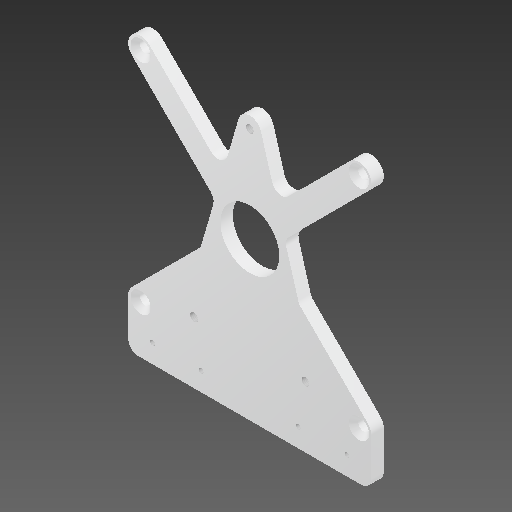
# Autodesk Inventor part: motor_support
Saved by Autodesk Inventor 2020.2 (Build 242310000, 310)
## iProperties
Created: 2020-03-23
Part Number: motor_support
Material: Aluminum 6061
Document SubType Name: Modeling
Designer: agmle
Density: 2.7 g/cm^3
Appearance: Aluminum - Flat
Mass: 160.03 g
Surface Area: 243.177 cm^2
Volume: 59.2703 cm^3
Author: agmle
Autodesk Inventor part; units mm, degrees
ref_plane "YZ Plane" through (0, 0, 0) normal (1, 0, 0) x (0, 1, 0)
ref_plane "XZ Plane" through (0, 0, 0) normal (0, 1, 0) x (-1, 0, 0)
ref_plane "XY Plane" through (0, 0, 0) normal (0, 0, 1) x (1, 0, 0)
sketch "Sketch1" plane through (0, 0, 0) normal (0, 0, 1) x (1, 0, 0)
  line L0 (36.3099, 124.6816) -> (0, 0)
  line L1 (0, 0) -> (72.6199, 0)
  line L2 (72.6199, 0) -> (36.3099, 124.6816)
  circle A0 centre (36.3099, 103.4017) radius 5.95 construction
  circle A1 centre (7.9299, 5.95) radius 5.95 construction
  circle A2 centre (64.6899, 5.95) radius 5.95 construction
  line L3 (36.3099, 103.4017) -> (7.9299, 5.95) construction
  line L4 (7.9299, 5.95) -> (64.6899, 5.95) construction
  line L5 (64.6899, 5.95) -> (36.3099, 103.4017) construction
  circle A3 centre (36.3098, 54.6757) radius 15
  line L6 (36.3099, 103.4017) -> (36.3098, 54.6757) construction
  line L7 (36.3098, 54.6757) -> (7.9299, 5.95) construction
  line L8 (36.3098, 54.6757) -> (64.6899, 5.95) construction
  point P0 (70.4026, 7.6137)
  dimension "d0" = 11.9
  dimension "d1" = 101.5
  dimension "d5" = 56.76
  dimension "d6" = 30
  dimension "d7" = 48.726
  dimension "d8" = 56.388
  constraints: 18 end point, 4 coincident, 4 tangent, 3 centre point, 2 horizontal, 1 equal length, 1 point on line, 6 other
  measures "d0" diameter of A0
  measures "d1" distance of L3.start L3.end
  measures "d5" distance of L3.end L4.end
  measures "d6" diameter of A3
  measures "d7" distance of L6.start L6.end
  measures "d8" distance of L6.end L7.end
extrude "Motor Mount" add sketch "Sketch1" along normal blind 6.35
fillet "Motor Edge Break" radius 5.95 3 edges at (36.3099, 124.6816, 3.175) (0, 0, 3.175) (72.6199, 0, 3.175)
sketch "Sketch2" plane through (0, 0, 6.35) normal (0, 0, 1) x (1, 0, 0)
  arc A0 (42.0226, 105.0653) -> (30.5973, 105.0653) centre (36.3099, 103.4017) ccw construction
  arc A1 (2.2173, 7.6137) -> (7.9299, 0) centre (7.9299, 5.95) ccw construction
  line L0 (36.3099, 103.4017) -> (7.9299, 5.95) construction
  line L1 (7.9299, 5.95) -> (64.6899, 5.95) construction
  line L2 (64.6899, 5.95) -> (36.3099, 103.4017) construction
  line L3 (7.9299, 0) -> (72.6199, 0) construction
  point P0 (0, 0)
  constraints: 6 end point, 3 coincident, 1 equal length, 1 parallel
hole "Motor Mount Bolts" at (36.3099, 103.4017, 6.35) at (7.9299, 5.95, 6.35) at (64.6899, 5.95, 6.35) direction (0, 0, -1) diameter 4.134 depth 14.1986 thread size "M5x0.8" class "6H" standard "ANSI Metric M Profile"
sketch "Sketch3" plane through (0, 0, 0) normal (0, 0, 1) x (1, 0, 0)
  circle A0 centre (36.3098, 54.6757) radius 15 construction
  circle A1 centre (36.3098, 54.6757) radius 72.39 construction
  line L0 (-19.3678, 110.3532) -> (91.9874, 110.3532) construction
  line L1 (91.9874, 110.3532) -> (91.9874, -1.0019) construction
  line L2 (91.9874, -1.0019) -> (-19.3678, -1.0019) construction
  line L3 (-19.3678, -1.0019) -> (-19.3678, 110.3532) construction
  line L4 (-19.3678, 110.3532) -> (91.9874, -1.0019) construction
  arc A2 (-14.8777, 114.8434) -> (-23.8579, 105.8631) centre (-19.3678, 110.3532) ccw
  line L5 (-23.8579, 105.8631) -> (18.4954, 63.5098)
  line L6 (30.5973, 105.0653) -> (2.2173, 7.6137) projected
  line L7 (22.5462, 77.4195) -> (-14.8777, 114.8434)
  line L8 (61.3841, 38.5816) -> (96.4775, 3.4882)
  line L9 (70.4026, 7.6137) -> (42.0226, 105.0653) projected
  line L10 (50.0736, 77.4197) -> (87.4973, 114.8434)
  line L11 (54.1244, 63.51) -> (96.4775, 105.8631)
  line L12 (11.2359, 38.582) -> (-23.8579, 3.4882)
  line L13 (3.8563, 13.2419) -> (-14.8777, -5.4921)
  arc A3 (-23.8579, 3.4882) -> (-14.8777, -5.4921) centre (-19.3678, -1.0019) ccw
  arc A4 (87.4973, -5.4921) -> (96.4775, 3.4882) centre (91.9874, -1.0019) ccw
  arc A5 (96.4775, 105.8631) -> (87.4973, 114.8434) centre (91.9874, 110.3532) ccw
  line L14 (68.7637, 13.2415) -> (87.4973, -5.4921)
  point P0 (0, 0)
  dimension "d19" = 144.78
  dimension "d20" = 12.7
  constraints: 26 end point, 9 point on line, 9 tangent, 8 point on circle, 6 coincident, 5 centre point, 4 collinear, 3 equal radius, 2 parallel, 2 perpendicular, 1 horizontal, 1 midpoint
  measures "d19" diameter of A1
  measures "d20" diameter of A2
extrude "Frame Legs" add sketch "Sketch3" along normal up to surface (6.35 mm away)
fillet "Frame Edge Break" radius 5 8 edges at (22.5462, 77.4195, 3.175) (50.0736, 77.4197, 3.175) (54.1244, 63.51, 3.175) (61.3841, 38.5816, 3.175) (11.2359, 38.582, 3.175) (18.4954, 63.5098, 3.175) (3.8563, 13.2419, 3.175) (68.7637, 13.2415, 3.175)
sketch "Sketch4" plane through (0, 0, 6.35) normal (0, 0, 1) x (1, 0, 0)
  arc A0 (-14.8777, 114.8434) -> (-23.8579, 105.8631) centre (-19.3678, 110.3532) ccw projected
  arc A1 (96.4775, 105.8631) -> (87.4973, 114.8434) centre (91.9874, 110.3532) ccw projected
  arc A2 (87.4973, -5.4921) -> (96.4775, 3.4882) centre (91.9874, -1.0019) ccw projected
  arc A3 (-23.8579, 3.4882) -> (-14.8777, -5.4921) centre (-19.3678, -1.0019) ccw projected
  point P0 (0, 0)
  constraints: 4 coincident
hole "Frame Mount Bolts" at (-19.3678, 110.3532, 6.35) at (91.9874, 110.3532, 6.35) at (91.9874, -1.0019, 6.35) at (-19.3678, -1.0019, 6.35) direction (0, 0, -1) diameter 5.5118 end through all countersink diameter 10.3886 countersink angle 90 clearance for "Flat Head Machine Screw" size "M5" standard "Ansi Metric M Profile"
sketch "Sketch5" plane through (0, 0, 6.35) normal (0, 0, 1) x (1, 0, 0)
  line L0 (-25.7178, -1.0019) -> (-25.7178, -25.4)
  line L1 (-25.7178, -25.4) -> (98.3374, -25.4)
  line L2 (98.3374, -25.4) -> (98.3374, -1.0019)
  arc A0 (-23.8579, 3.4882) -> (-14.8777, -5.4921) centre (-19.3678, -1.0019) ccw projected
  arc A1 (87.4973, -5.4921) -> (96.4775, 3.4882) centre (91.9874, -1.0019) ccw projected
  line L3 (7.9299, 0) -> (64.6899, 0) projected
  arc A2 (2.7209, 3.0745) -> (7.9299, 0) centre (7.9299, 5.95) ccw projected
  arc A3 (2.7209, 3.0745) -> (-5.192, 4.1936) centre (-1.6564, 0.6581) ccw projected
  line L4 (-5.192, 4.1936) -> (-14.8777, -5.4921) projected
  arc A4 (64.6899, 0) -> (69.8989, 3.0744) centre (64.6899, 5.95) ccw projected
  arc A5 (77.8117, 4.1935) -> (69.8989, 3.0744) centre (74.2762, 0.6579) ccw projected
  line L5 (87.4973, -5.4921) -> (77.8117, 4.1935) projected
  point P0 (0, 0)
  dimension "d31" = 25.4
  constraints: 6 end point, 2 perpendicular, 2 point on circle, 2 tangent, 1 vertical
  measures "d31" distance between parallel lines of L3 L1
extrude "Support Mount" add sketch "Sketch5" against normal up to surface (6.35 mm away)
fillet "Support Edge Break" radius 5 2 edges at (-25.7178, -25.4, 3.175) (98.3374, -25.4, 3.175)
sketch "Sketch6" plane through (0, 0, 6.35) normal (0, 0, 1) x (1, 0, 0)
  line L0 (-13.2202, -15.875) -> (11.5448, -15.875) construction
  line L1 (11.5448, -15.875) -> (36.3098, -15.875) construction
  line L2 (36.3098, -15.875) -> (61.0748, -15.875) construction
  line L3 (61.0748, -15.875) -> (85.8398, -15.875) construction
  line L4 (-20.7178, -25.4) -> (93.3374, -25.4) construction
  line L5 (-25.7178, -1.0019) -> (-25.7178, -20.4) construction
  line L6 (93.3374, -25.4) -> (-20.7178, -25.4) construction
  line L7 (36.3098, -25.4) -> (36.3098, -15.875) construction
  circle A0 centre (36.3098, 54.6757) radius 15 projected
  point P0 (0, 0)
  dimension "d36" = 9.525
  dimension "d44" = 24.765
  dimension "d45" = 70.5507
  constraints: 10 end point, 6 collinear, 1 midpoint, 1 parallel, 1 perpendicular
  measures "d36" distance of L7.start L1.end
  measures "d44" distance of L0.start L0.end
  measures "d45" distance of L1.end A0.centre
hole "Support Mount Bolts" at (-13.2202, -15.875, 6.35) at (11.5448, -15.875, 6.35) at (61.0748, -15.875, 6.35) at (85.8398, -15.875, 6.35) direction (0, 0, -1) diameter 2.459 end through all thread size "M3x0.5" class "6H" standard "ANSI Metric M Profile"
equation "\"d19\" = 2 * drum_radius + 2 * drum_wall_height"
equation "\"drum_radius\" = 59.69"
equation "\"drum_wall_height\" = 12.7"
body "Solid1"
